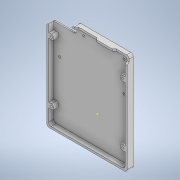
# Autodesk Inventor part: base
Saved by Autodesk Inventor 2021 (Build 250183000, 183)
## iProperties
Created: 2023-07-02
Part Number: base
Material: Generic
Document SubType Name: Modeling
Designer: Toby
Density: 1 g/cm^3
Appearance: Default
Author: Toby
Autodesk Inventor part; units mm, degrees
ref_plane "YZ Plane" through (0, 0, 0) normal (1, 0, 0) x (0, 1, 0)
ref_plane "XZ Plane" through (0, 0, 0) normal (0, 1, 0) x (-1, 0, 0)
ref_plane "XY Plane" through (0, 0, 0) normal (0, 0, 1) x (1, 0, 0)
sketch "Sketch1" plane through (0, 0, 0) normal (0, 0, 1) x (1, 0, 0)
  line L0 (-45.4294, 68.478) -> (34.5706, 68.478)
  line L1 (34.5706, 68.478) -> (34.5706, -30.822)
  line L2 (34.5706, -30.822) -> (-45.4294, -30.822)
  line L3 (-45.4294, -30.822) -> (-45.4294, 68.478)
  line L4 (-43.4294, 66.478) -> (32.5706, 66.478)
  line L5 (32.5706, 66.478) -> (32.5706, -28.822)
  line L6 (32.5706, -28.822) -> (-43.4294, -28.822)
  line L7 (-43.4294, -28.822) -> (-43.4294, 66.478)
  point P0 (0, 0)
  dimension "d0" = 80
  dimension "d1" = 99.3
  dimension "d2" = 2
  dimension "d3" = 2
  dimension "d4" = 2
  dimension "d5" = 2
  constraints: 16 end point, 4 parallel, 2 horizontal, 2 perpendicular
  measures "d0" distance of L0.start L0.end
  measures "d1" distance of L2.end L0.start
  measures "d2" distance between parallel lines of L0 L4
  measures "d3" distance between parallel lines of L2 L6
  measures "d4" distance between parallel lines of L3 L7
  measures "d5" distance between parallel lines of L1 L5
extrude "Extrusion1" add sketch "Sketch1" along normal blind 5
fillet "Fillet1" radius 2.5 8 edges at (-43.4294, 66.478, 2.5) (-45.4294, 68.478, 2.5) (32.5706, 66.478, 2.5) (34.5706, 68.478, 2.5) (-43.4294, -28.822, 2.5) (-45.4294, -30.822, 2.5) (34.5706, -30.822, 2.5) (32.5706, -28.822, 2.5)
sketch "Sketch2" plane through (0, 0, 5) normal (0, 0, 1) x (1, 0, 0)
  line L0 (-45.4294, 65.978) -> (-45.4294, -28.322) projected
  line L1 (-42.9294, -30.822) -> (32.0706, -30.822) projected
  line L2 (-43.4294, -26.322) -> (-43.4294, 63.978) projected
  line L3 (-43.4294, 50.926) -> (-38.2294, 50.926)
  line L4 (-38.2294, 50.926) -> (-38.2294, 45.926)
  line L5 (-38.2294, 45.926) -> (-43.4294, 45.926)
  line L6 (-43.4294, 45.926) -> (-43.4294, 50.926)
  line L7 (32.5706, 63.978) -> (32.5706, -26.322) projected
  line L8 (32.5706, 50.799) -> (27.6306, 50.799)
  line L9 (27.6306, 50.799) -> (27.6306, 45.799)
  line L10 (27.6306, 45.799) -> (32.5706, 45.799)
  line L11 (32.5706, 45.799) -> (32.5706, 50.799)
  line L12 (-43.4294, -9.022) -> (-38.2294, -9.022)
  line L13 (-38.2294, -9.022) -> (-38.2294, -14.022)
  line L14 (-38.2294, -14.022) -> (-43.4294, -14.022)
  line L15 (-43.4294, -14.022) -> (-43.4294, -9.022)
  line L16 (32.5706, -9.022) -> (27.6306, -9.022)
  line L17 (27.6306, -9.022) -> (27.6306, -14.022)
  line L18 (27.6306, -14.022) -> (32.5706, -14.022)
  line L19 (32.5706, -14.022) -> (32.5706, -9.022)
  circle A0 centre (-40.7294, 48.426) radius 1
  circle A1 centre (30.1306, 48.299) radius 1
  circle A2 centre (-40.7294, -11.522) radius 1
  circle A3 centre (30.1306, -11.622) radius 1
  point P0 (0, 0)
  dimension "d9" = 4.7
  dimension "d10" = 19.3
  dimension "d11" = 19.2
  dimension "d12" = 75.56
  dimension "d13" = 79.248
  dimension "d14" = 4.7
  dimension "d15" = 79.121
  dimension "d16" = 75.56
  dimension "d17" = 5
  dimension "d18" = 2.5
  dimension "d19" = 2.5
  dimension "d20" = 5
  dimension "d21" = 2.5
  dimension "d22" = 2.5
  dimension "d23" = 2.5
  dimension "d24" = 2.5
  dimension "d25" = 2.5
  dimension "d26" = 2.5
  dimension "d27" = 2
  dimension "d28" = 2
  dimension "d29" = 2
  dimension "d30" = 2
  constraints: 32 end point, 8 parallel, 6 point on line, 4 centre point, 4 coincident, 4 horizontal, 4 perpendicular
  measures "d9" distance from line of L0 point (-40.729, -11.522)
  measures "d10" distance from line of L1 point (-40.729, -11.522)
  measures "d11" distance from line of L1 point (30.131, -11.622)
  measures "d12" distance from line of L0 point (30.131, -11.622)
  measures "d13" distance from line of L1 point (-40.729, 48.426)
  measures "d14" distance from line of L0 point (-40.729, 48.426)
  measures "d15" distance from line of L1 point (30.131, 48.299)
  measures "d16" distance from line of L0 point (30.131, 48.299)
  measures "d17" distance between parallel lines of L5 L3
  measures "d18" distance from line of L3 point (-40.729, 48.426)
  measures "d19" distance from line of L4 point (-40.729, 48.426)
  measures "d20" distance of L8.end L9.end
  measures "d21" distance from line of L8 point (30.131, 48.299)
  measures "d22" distance from line of L9 point (30.131, 48.299)
  measures "d23" distance from line of point (-40.729, -11.522) L12
  measures "d24" distance from line of L14 point (-40.729, -11.522)
  measures "d25" distance from line of point (-40.729, -11.522) L13
  measures "d26" distance from line of point (30.131, -11.622) L17
  measures "d27" diameter of A0
  measures "d28" diameter of A1
  measures "d29" diameter of A2
  measures "d30" diameter of A3
extrude "Extrusion2" add sketch "Sketch2" against normal blind 5
fillet "Fillet2" radius 2.5 8 edges at (-38.2294, -14.022, 2.5) (-38.2294, -9.022, 2.5) (27.6306, -14.022, 2.5) (27.6306, -9.022, 2.5) (27.6306, 45.799, 2.5) (27.6306, 50.799, 2.5) (-38.2294, 45.926, 2.5) (-38.2294, 50.926, 2.5)
sketch "Sketch9" plane through (0, 0, 0) normal (0, 0, -1) x (-1, 0, 0)
  line L0 (-34.5706, -30.822) -> (45.4294, -30.822)
  line L1 (45.4294, -30.822) -> (45.4294, 68.478)
  line L2 (45.4294, 68.478) -> (-34.5706, 68.478)
  line L3 (-34.5706, 68.478) -> (-34.5706, -30.822)
  line L4 (-34.5706, -28.322) -> (-34.5706, 65.978) projected
  line L5 (42.9294, -30.822) -> (-32.0706, -30.822) projected
  line L6 (45.4294, 65.978) -> (45.4294, -28.322) projected
  line L7 (-32.0706, 68.478) -> (42.9294, 68.478) projected
  point P0 (0, 0)
  constraints: 8 end point, 4 collinear, 2 parallel, 1 horizontal, 1 perpendicular
extrude "Extrusion8" add sketch "Sketch9" along normal blind 1.2
sketch "Sketch7" plane through (0, 0, 5) normal (0, 0, 1) x (1, 0, 0)
  line L0 (-20.4294, 68.478) -> (34.5706, 68.478)
  line L1 (34.5706, 68.478) -> (34.5706, 63.478)
  line L2 (34.5706, 63.478) -> (-20.4294, 63.478)
  line L3 (-20.4294, 63.478) -> (-20.4294, 68.478)
  line L4 (32.0706, 68.478) -> (-42.9294, 68.478) projected
  line L5 (-20.4294, 65.978) -> (-20.4294, 60.9804) projected
  line L6 (34.5706, -28.322) -> (34.5706, 65.978) projected
  point P0 (0, 0)
  point P1 (-17.9294, 68.478)
  dimension "d52" = 5
  constraints: 8 end point, 3 collinear, 2 parallel, 1 horizontal, 1 perpendicular
  measures "d52" distance between parallel lines of L0 L2
extrude "Extrusion7" cut sketch "Sketch7" against normal blind 2
chamfer "Chamfer1" distance 2 angle 45 1 edges at (33.5706, 63.478, 5)
sketch "Sketch8" plane through (0, 0, 0) normal (0, 0, -1) x (-1, 0, 0)
  point P0 (0, 0)
fillet "Fillet5" radius 2.5 4 edges at (34.5706, -30.822, -0.6) (34.5706, 68.478, -0.6) (-45.4294, 68.478, -0.6) (-45.4294, -30.822, -0.6)
sketch "Sketch10" plane through (0, 0, -1.2) normal (0, 0, -1) x (-1, 0, 0)
  line L0 (20.4294, 68.478) -> (45.4294, 68.478)
  line L1 (45.4294, 68.478) -> (45.4294, 58.478)
  line L2 (45.4294, 58.478) -> (20.4294, 58.478)
  line L3 (20.4294, 58.478) -> (20.4294, 68.478)
  line L4 (42.9294, 68.478) -> (-32.0706, 68.478) projected
  line L5 (45.4294, -28.322) -> (45.4294, 65.978) projected
  point P0 (0, 0)
  dimension "d61" = 10
  dimension "d62" = 25
  constraints: 8 end point, 2 collinear, 2 parallel, 1 horizontal, 1 perpendicular
  measures "d61" distance between parallel lines of L2 L4
  measures "d62" distance between parallel lines of L5 L3
extrude "Extrusion9" cut sketch "Sketch10" against normal blind 30
fillet "Fillet6" radius 2.5 3 edges at (-20.4294, 68.478, 0.9) (-45.4294, 58.478, 1.9) (-20.4294, 58.478, -0.6)
sketch "Sketch11" plane through (0, 0, -1.2) normal (0, 0, -1) x (-1, 0, 0)
  line L0 (17.9294, 68.478) -> (-32.0706, 68.478) projected
  line L1 (-34.5706, 65.978) -> (-34.5706, -28.322) projected
  line L2 (45.4294, -28.322) -> (45.4294, 55.978) projected
  point P0 (0, 0)
  point P1 (-26.5706, 60.478)
  point P2 (-26.5706, 30.478)
  point P3 (37.4294, 30.478)
  point P4 (13.4294, 60.478)
  dimension "d66" = 8
  dimension "d67" = 8
  dimension "d68" = 8
  dimension "d69" = 8
  dimension "d70" = 30
  dimension "d71" = 30
  dimension "d72" = 8
  dimension "d73" = 40
  measures "d66" distance from line of L0 point (-26.571, 60.478)
  measures "d67" distance from line of L1 point (-26.571, 60.478)
  measures "d68" distance from line of L1 point (-26.571, 30.478)
  measures "d69" distance from line of L2 point (37.429, 30.478)
  measures "d70" distance of point (-26.571, 60.478) point (-26.571, 30.478)
  measures "d71" vertical distance of point (37.429, 30.478) point (-26.571, 60.478)
  measures "d72" distance from line of L0 point (13.429, 60.478)
  measures "d73" distance of point (-26.571, 60.478) point (13.429, 60.478)
hole "Hole1" at (26.5706, 60.478, -1.2) at (26.5706, 30.478, -1.2) at (-37.4294, 30.478, -1.2) at (-13.4294, 60.478, -1.2) direction (0, 0, 1) diameter 2 depth 8 tip angle 118
sketch "Sketch12" plane through (0, 0, 3) normal (0, 0, 1) x (1, 0, 0)
  line L0 (-20.3789, 66.478) -> (30.0706, 66.478) projected
  line L1 (-17.9294, 68.478) -> (32.0706, 68.478) projected
  line L2 (-20.3789, 66.478) -> (-15.3789, 66.478)
  line L3 (-15.3789, 66.478) -> (-15.3789, 68.478)
  line L4 (-15.3789, 68.478) -> (-20.3789, 68.478)
  line L5 (-20.3789, 68.478) -> (-20.3789, 66.478)
  line L6 (4.5706, 66.478) -> (19.5706, 66.478)
  line L7 (19.5706, 66.478) -> (19.5706, 68.478)
  line L8 (19.5706, 68.478) -> (4.5706, 68.478)
  line L9 (4.5706, 68.478) -> (4.5706, 66.478)
  line L10 (34.5706, -28.322) -> (34.5706, 61.478) projected
  point P0 (0, 0)
  point P1 (4.5706, 68.478)
  dimension "d81" = 5
  dimension "d82" = 15
  dimension "d83" = 30
  constraints: 16 end point, 4 parallel, 3 point on line, 2 horizontal, 2 perpendicular
  measures "d81" distance between parallel lines of L3 L5
  measures "d82" distance between parallel lines of L10 L7
  measures "d83" distance from line of L10 L6.start
extrude "Extrusion10" add sketch "Sketch12" along normal blind 2 contours L5 L4 L1 L3 L0 | L9 L1 L7 L0
chamfer "Chamfer2" distance 2 angle 45 2 edges at (19.5706, 67.478, 3) (4.5706, 67.478, 3)
chamfer "Chamfer3" distance 2 angle 45 1 edges at (-15.3789, 67.478, 5)
fillet "Fillet7" radius 2.5 1 edges at (-20.3789, 68.478, 4)
body "Solid1"
